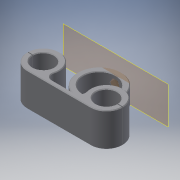
# Autodesk Inventor part: PlotterPenHolder
Saved by Autodesk Inventor 2018 (Build 220112000, 112)
## iProperties
Created: 2018-05-11
Part Number: PlotterPenHolder
Material: Generic
Document SubType Name: Modeling
Designer: Jasper
Density: 1 g/cm^3
Appearance: Default
Author: Jasper
Autodesk Inventor part; units mm, degrees
ref_plane "YZ Plane" through (0, 0, 0) normal (1, 0, 0) x (0, 1, 0)
ref_plane "XZ Plane" through (0, 0, 0) normal (0, 1, 0) x (-1, 0, 0)
ref_plane "XY Plane" through (0, 0, 0) normal (0, 0, 1) x (1, 0, 0)
sketch "Sketch1" plane through (0, 0, 0) normal (0, 0, 1) x (1, 0, 0)
  circle A0 centre (0, 0) radius 7.5265
  line L0 (0, 0) -> (-45.153, 0) construction
  line L1 (-22.5765, 0) -> (-22.5765, 19.7595) construction
  circle A1 centre (0, 0) radius 11.5
  circle A2 centre (-45.153, 0) radius 7.5265
  circle A3 centre (-45.153, 0) radius 11.5
  dimension "d0" = 15.053
  dimension "d1" = 45.153
  dimension "d2" = 23
  constraints: 4 centre point, 4 coincident, 4 end point, 2 symmetric about line, 1 horizontal, 1 midpoint, 1 vertical, 2 other
  measures "d0" diameter of A0
  measures "d1" distance of L0.start L0.end
  measures "d2" diameter of A1
extrude "Extrusion1" add sketch "Sketch1" against normal blind 24
sketch "Sketch2" plane through (0, 0, 0) normal (0, 0, 1) x (1, 0, 0)
  circle A0 centre (0, 0) radius 11.5 projected
  line L0 (0, -11.5) -> (-45.153, -11.5)
  circle A1 centre (-45.153, 0) radius 11.5 projected
  line L1 (-7.746, -8.5) -> (-37.407, -8.5)
  line L2 (0, 0) -> (0, -11.5) construction
  line L3 (-45.153, 0) -> (-45.153, -11.5) construction
  dimension "d5" = 3
  constraints: 8 end point, 5 point on circle, 2 horizontal, 1 parallel, 1 vertical
  measures "d5" distance between parallel lines of L1 L0
extrude "Extrusion2" add sketch "Sketch2" against normal up to surface (24 mm away) contours A0 L0 A1 L1
sketch "Sketch4" plane through (0, 0, -24) normal (0, 0, -1) x (-1, 0, 0)
  line L0 (7.746, -8.5) -> (37.407, -8.5) construction
  line L1 (7.746, -8.5) -> (37.407, -8.5) construction
  line L2 (22.5765, -8.5) -> (22.5765, 17.5) construction
  circle A0 centre (22.5765, 17.5) radius 11.5
  circle A1 centre (22.5765, 17.5) radius 15.5
  arc A2 (7.746, -8.5) -> (0, -11.5) centre (0, 0) ccw projected
  line L3 (37.407, -8.5) -> (7.746, -8.5) projected
  line L4 (20.0765, -8.5) -> (20.0765, 2.2029)
  line L5 (25.0765, -8.5) -> (25.0765, 2.2029)
  dimension "d9" = 23
  dimension "d10" = 4
  dimension "d11" = 5
  dimension "d13" = 26
  constraints: 8 end point, 2 centre point, 2 perpendicular, 2 point on circle, 2 point on line, 1 coincident, 1 horizontal, 1 midpoint, 1 parallel, 1 other
  measures "d9" diameter of A0
  measures "d10" radial gap between concentric circles of A0 A1
  measures "d11" distance between parallel lines of L5 L4
  measures "d13" distance of L2.start L2.end
extrude "Extrusion3" add sketch "Sketch4" against normal blind 12
ref_plane "Work Plane2" through (-22.5765, 29, -24) normal (0, -1, 0) x (1, 0, 0)
sketch "Sketch5" plane through (-22.5765, 29, -24) normal (0, -1, 0) x (1, 0, 0)
  line L0 (15.5, 12) -> (-15.5, 12) projected
  line L1 (-15.5, 0) -> (15.5, 0) projected
  line L2 (-11.5, 12) -> (11.5, 12) construction
  line L3 (0, 12) -> (0, 0) construction
  line L4 (11.5, 0) -> (-11.5, 0) construction
  line L5 (1.8764, 9.25) -> (3.7528, 6)
  line L6 (3.7528, 6) -> (1.8764, 2.75)
  line L7 (1.8764, 2.75) -> (-1.8764, 2.75)
  line L8 (-1.8764, 2.75) -> (-3.7528, 6)
  line L9 (-3.7528, 6) -> (-1.8764, 9.25)
  line L10 (-1.8764, 9.25) -> (1.8764, 9.25)
  point P0 (22.5765, 24)
  point P1 (2.5, 12)
  point P2 (-2.5, 12)
  point P3 (-2.5, 0)
  point P4 (2.5, 0)
  point P5 (0, 6)
  point P6 (0, 9.25)
  dimension "d16" = 6.5
  constraints: 14 end point, 4 midpoint, 1 point on line, 13 other
  measures "d16" distance between parallel lines of L7 L10
extrude "Extrusion4" cut sketch "Sketch5" along normal blind 1 and the other way blind 3.1
sketch "Sketch6" plane through (-22.5765, 32.1, -24) normal (0, -1, 0) x (1, 0, 0)
  line L0 (1.8764, 2.75) -> (-1.8764, 2.75) projected
  line L1 (1.8764, 2.75) -> (-1.8764, 2.75) projected
  line L2 (-1.8764, 9.25) -> (1.8764, 9.25) construction
  line L3 (0, 9.25) -> (0, 2.75) construction
  circle A0 centre (0, 6) radius 1.75
  point P0 (22.5765, 24)
  dimension "d21" = 3.5
  constraints: 3 midpoint, 2 end point, 1 centre point
  measures "d21" diameter of A0
extrude "Extrusion5" cut sketch "Sketch6" against normal through all
fillet "Fillet1" radius 4 4 edges at (-20.0765, -8.5, -18) (-25.0765, -8.5, -18) (-25.0765, 2.2029, -18) (-20.0765, 2.2029, -18)
fillet "Fillet2" radius 4 2 edges at (-7.746, -8.5, -12) (-37.407, -8.5, -12)
fillet "Fillet3" radius 4 1 edges at (-22.5765, -8.5, -12)
chamfer "Chamfer1" distance 0.5 angle 45 32 edges at (-7.5265, 0, 0) (6.8504, 9.237, 0) (-22.5765, -11.5, 0) (-52.0034, 9.237, 0) (-33.5335, -6.8827, 0) (-22.5765, -8.5, 0) (-11.6195, -6.8827, 0) (-52.6795, 0, 0) (-22.5765, -11.5, -24) (-52.0034, 9.237, -24) (-33.5335, -6.8827, -24) (-29.6986, -8.5, -24) (-26.2481, -7.3284, -24) (-25.0765, -2.6924, -24) (-25.8105, 1.4246, -24) (-22.5765, 33, -24) (-19.3425, 1.4246, -24) (-20.0765, -2.6924, -24) (-18.9049, -7.3284, -24) (-15.4544, -8.5, -24) (-11.6195, -6.8827, -24) (6.8504, 9.237, -24) (-7.5265, 0, -24) (-11.0765, 17.5, -24) (-11.0765, 17.5, -12) (-22.5765, 33, -12) (-25.8105, 1.4246, -12) (-25.0765, -2.6924, -12) (-26.2481, -7.3284, -10.8284) (-19.3425, 1.4246, -12) (-20.0765, -2.6924, -12) (-18.9049, -7.3284, -10.8284)
sketch "Sketch7" plane through (0, 0, 0) normal (0, 0, 1) x (1, 0, 0)
  line L0 (-11.5, 0.25) -> (11.5, 0.25)
  line L1 (11.5, 0.25) -> (11.5, -0.25)
  line L2 (11.5, -0.25) -> (-11.5, -0.25)
  line L3 (-11.5, -0.25) -> (-11.5, 0.25)
  line L4 (-11.5, 0.25) -> (11.5, -0.25) construction
  line L5 (11.5, 0.25) -> (-11.5, -0.25) construction
  arc A0 (0, -11.5) -> (-11.0047, -3.3387) centre (0, 0) ccw projected
  line L6 (0, -0.25) -> (0, 0.25)
  line L7 (0, -11.5) -> (-45.153, -11.5) construction
  line L8 (-22.5765, -11.5) -> (-22.5765, 33) construction
  arc A1 (-17.4098, 2.8865) -> (-27.7432, 2.8865) centre (-22.5765, 17.5) ccw construction
  line L9 (-33.653, 0.25) -> (-56.653, 0.25)
  line L10 (-56.653, 0.25) -> (-56.653, -0.25)
  line L11 (-56.653, -0.25) -> (-33.653, -0.25)
  line L12 (-33.653, -0.25) -> (-33.653, 0.25)
  line L13 (-33.653, 0.25) -> (-56.653, -0.25) construction
  line L14 (-56.653, 0.25) -> (-33.653, -0.25) construction
  line L15 (-45.153, -0.25) -> (-45.153, 0.25)
  point P0 (-45.153, 0)
  point P1 (-34.1483, -3.3387)
  point P2 (-45.153, 0)
  dimension "d30" = 0.5
  constraints: 30 end point, 9 symmetric about line, 7 midpoint, 2 parallel, 1 horizontal, 1 perpendicular, 1 point on circle, 1 tangent, 1 vertical
  measures "d30" distance between parallel lines of L0 L2
extrude "Extrusion6" cut sketch "Sketch7" against normal through all contours L0 A0 L2 L6 | L0 L1 A0 | L1 L2 A0 | L15 L11 L10 L9 picked at (3.8333, 0)
sketch "Sketch8" plane through (0, 0, -12) normal (0, 0, 1) x (1, 0, 0)
  line L0 (-20.0765, -4.5) -> (-25.0765, -4.5) construction
  line L1 (-20.0765, -4.5) -> (-25.0765, -4.5) construction
  line L2 (-22.5765, -4.5) -> (-22.5765, -3.5) construction
  line L3 (-20.0765, -3) -> (-25.0765, -3)
  line L4 (-25.0765, -3) -> (-25.0765, -4)
  line L5 (-25.0765, -4) -> (-20.0765, -4)
  line L6 (-20.0765, -4) -> (-20.0765, -3)
  line L7 (-20.0765, -3) -> (-25.0765, -4) construction
  line L8 (-25.0765, -3) -> (-20.0765, -4) construction
  line L9 (-20.0765, -4.5) -> (-20.0765, -0.8848) projected
  point P0 (0, 0)
  dimension "d33" = 1
  dimension "d34" = 1
  constraints: 16 end point, 3 midpoint, 2 horizontal, 2 parallel, 1 collinear, 1 perpendicular, 1 vertical
  measures "d33" distance between parallel lines of L3 L5
  measures "d34" distance of L2.start L2.end
extrude "Extrusion7" cut sketch "Sketch8" against normal blind 2
fillet "Fillet4" radius 2 2 edges at (-25.0765, -3.5, -14) (-20.0765, -3.5, -14)
fillet "Fillet5" radius 2 2 edges at (-22.5765, -3, -12) (-22.5765, -4, -12)
body "Solid1"
